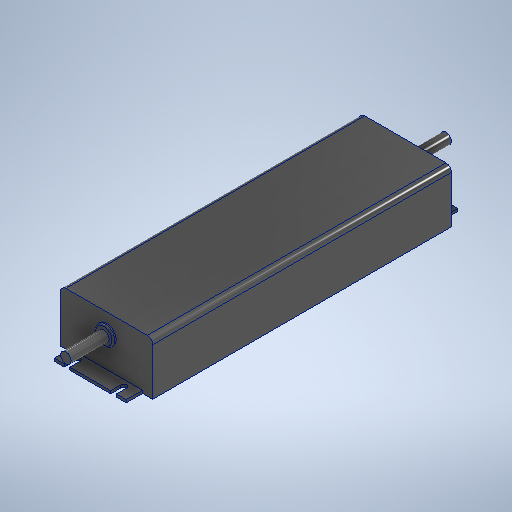
# Autodesk Inventor part: HEP-240-24A
Saved by Autodesk Inventor 2025 (Build 290162000, 162)
## iProperties
Created: 2024-06-10
Part Number: HEP-240-24A
Material: Generic
Document SubType Name: Modeling
Designer: Caleb Fangmeier
Density: 1 g/cm^3
Appearance: Aluminum - Flat
Author: Caleb Fangmeier
Autodesk Inventor part; units mm, degrees
ref_plane "YZ Plane" through (0, 0, 0) normal (1, 0, 0) x (0, 1, 0)
ref_plane "XZ Plane" through (0, 0, 0) normal (0, 1, 0) x (-1, 0, 0)
ref_plane "XY Plane" through (0, 0, 0) normal (0, 0, 1) x (1, 0, 0)
sketch "Sketch1" plane through (0, 0, 0) normal (0, 1, 0) x (-1, 0, 0)
  line L0 (26.5, -122.1) -> (26.5, 122.1)
  line L1 (-26.5, 122.1) -> (-26.5, -122.1)
  line L2 (-26.5, -122.1) -> (26.5, 122.1) construction
  line L3 (26.5, -122.1) -> (-26.5, 122.1) construction
  line L4 (15, 122.1) -> (15, 114.6)
  line L5 (17.1, 112.5) -> (17.1, 112.5)
  line L6 (19.2, 114.6) -> (19.2, 122.1)
  line L7 (26.5, 122.1) -> (19.2, 122.1)
  arc A0 (17.1, 112.5) -> (19.2, 114.6) centre (17.1, 114.6) ccw
  arc A1 (15, 114.6) -> (17.1, 112.5) centre (17.1, 114.6) ccw
  line L8 (15, 122.1) -> (0, 122.1)
  line L9 (0, 145.2544) -> (0, -156.3488)
  line L10 (57.515, 0) -> (-80.9383, 0)
  line L11 (26.5, -122.1) -> (-26.5, 122.1) construction
  line L12 (-15, 122.1) -> (-15, 114.6)
  line L13 (-17.1, 112.5) -> (-17.1, 112.5)
  line L14 (-19.2, 114.6) -> (-19.2, 122.1)
  line L15 (-26.5, 122.1) -> (-19.2, 122.1)
  arc A2 (-19.2, 114.6) -> (-17.1, 112.5) centre (-17.1, 114.6) ccw
  arc A3 (-17.1, 112.5) -> (-15, 114.6) centre (-17.1, 114.6) ccw
  line L16 (-15, 122.1) -> (0, 122.1)
  line L17 (-26.5, 122.1) -> (26.5, -122.1) construction
  line L18 (26.5, 122.1) -> (-26.5, -122.1) construction
  line L19 (15, -122.1) -> (15, -114.6)
  line L20 (19.2, -114.6) -> (19.2, -122.1)
  line L21 (26.5, -122.1) -> (19.2, -122.1)
  arc A4 (19.2, -114.6) -> (17.1, -112.5) centre (17.1, -114.6) ccw
  arc A5 (17.1, -112.5) -> (15, -114.6) centre (17.1, -114.6) ccw
  line L22 (15, -122.1) -> (0, -122.1)
  line L23 (0, -145.2544) -> (0, 156.3488)
  line L24 (26.5, 122.1) -> (-26.5, -122.1) construction
  arc A6 (-15, -114.6) -> (-17.1, -112.5) centre (-17.1, -114.6) ccw
  line L25 (-15, -122.1) -> (-15, -114.6)
  line L26 (-19.2, -114.6) -> (-19.2, -122.1)
  line L27 (-26.5, -122.1) -> (-19.2, -122.1)
  line L28 (-15, -122.1) -> (0, -122.1)
  arc A7 (-17.1, -112.5) -> (-19.2, -114.6) centre (-17.1, -114.6) ccw
  point P0 (0, 0)
  point P1 (0, 0)
  point P2 (0, 0)
  point P3 (-17.1, -112.5)
  point P4 (17.1, -112.5)
  point P5 (17.1, 112.5)
  dimension "d0" = 244.2
  dimension "d1" = 53
  dimension "d2" = 9.6
  dimension "d3" = 2.1
  dimension "d4" = 9.4
  dimension "d5" = 4.2
  constraints: 58 end point, 31 symmetric about line, 16 point on circle, 8 centre point, 4 midpoint, 4 tangent, 3 horizontal, 3 parallel, 2 horizontal alignment, 2 point on line, 1 concentric, 1 perpendicular, 1 vertical, 1 vertical alignment, 6 other
  measures "d0" distance of L0.start L0.end
  measures "d1" distance of L0.end L1.start
  measures "d2" distance between parallel lines of L7 L5
  measures "d3" radius of A0
  measures "d4" distance from line of L0 A0.centre
  measures "d5" distance between parallel lines of L6 L4
extrude "Extrusion1" add sketch "Sketch1" along normal blind 2
sketch "Sketch2" plane through (0, 0, 0) normal (0, -1, 0) x (1, 0, 0)
  line L0 (-34, -110.1) -> (34, -110.1)
  line L1 (34, -110.1) -> (34, 110.1)
  line L2 (34, 110.1) -> (-34, 110.1)
  line L3 (-34, 110.1) -> (-34, -110.1)
  line L4 (-34, -110.1) -> (34, 110.1) construction
  line L5 (34, -110.1) -> (-34, 110.1) construction
  point P0 (0, 0)
  dimension "d8" = 220.2
  dimension "d9" = 68
  constraints: 12 end point, 2 midpoint, 2 parallel, 1 horizontal, 1 perpendicular
  measures "d8" distance of L0.end L1.end
  measures "d9" distance of L1.end L2.end
extrude "Extrusion2" add sketch "Sketch2" against normal blind 38.8
fillet "Fillet1" radius 4 2 edges at (34, 38.8, 0) (-34, 38.8, 0)
sketch "Sketch3" plane through (34, 0, -110.1) normal (0, 0, -1) x (-1, 0, 0)
  circle A0 centre (34, 24.5) radius 7.1
  circle A1 centre (34, 24.5) radius 3.9
  line L0 (19, 0) -> (49, 0) projected
  point P0 (34, 0)
  point P1 (34, 0)
  dimension "d13" = 24.5
  dimension "d14" = 14.2
  dimension "d15" = 7.8
  constraints: 2 centre point, 1 coincident, 1 midpoint, 1 vertical alignment
  measures "d13" distance from line of L0 A0.centre
  measures "d14" diameter of A0
  measures "d15" diameter of A1
extrude "Extrusion3" add sketch "Sketch3" along normal blind 2 contours A0 | A1
extrude "Extrusion4" add sketch "Sketch3" along normal blind 30 contours A1
fillet "Fillet2" radius 1 1 edges at (7.1, 24.5, -112.1)
mirror "Mirror1" about plane through (0, 0, 0) normal (0, 0, 1) of "Extrusion3", "Extrusion4", "Fillet2"
equation "\"d5\" = 2 * d3"
body "Solid1"
